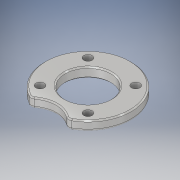
# Autodesk Inventor part: Motor Mount
Saved by Autodesk Inventor 2019.4 (Build 234330000, 330)
## iProperties
Created: 2019-03-01
Part Number: Motor Mount
Material: Aluminum 6061-AHC
Document SubType Name: Modeling
Designer: Petar
Density: 2.7 g/cm^3
Appearance: Aluminum - Dark
Mass: 6.25091 g
Surface Area: 19.0882 cm^2
Volume: 2.31515 cm^3
Author: Petar
Autodesk Inventor part; units mm, degrees
ref_plane "YZ Plane" through (0, 0, 0) normal (1, 0, 0) x (0, 1, 0)
ref_plane "XZ Plane" through (0, 0, 0) normal (0, 1, 0) x (-1, 0, 0)
ref_plane "XY Plane" through (0, 0, 0) normal (0, 0, 1) x (1, 0, 0)
sketch "Sketch1" plane through (0, 0, 0) normal (0, 1, 0) x (-1, 0, 0)
  circle A0 centre (0, 0) radius 9.25
  circle A1 centre (0, 0) radius 13.75 construction
  circle A2 centre (9.7227, -9.7227) radius 1.7
  line L0 (9.7227, -9.7227) -> (0, 0) construction
  circle A3 centre (9.7227, 9.7227) radius 1.7
  circle A4 centre (-9.7227, 9.7227) radius 1.7
  circle A5 centre (-9.7227, -9.7227) radius 1.7
  line L1 (0, 0) -> (0, -13.75) construction
  circle A6 centre (0, 0) radius 17.5
  circle A7 centre (0, 0) radius 10 construction
  line L2 (7.5, 15.8114) -> (0, 10) construction
  line L3 (0, 10) -> (-7.5, 15.8114) construction
  spline S0 degree 2 poles (7.5, 15.8114) (0, 10) (-7.5, 15.8114) knots 1 1 1 2 2 2
  line L4 (7.5, 15.8114) -> (-7.5, 15.8114) construction
  line L5 (0, 10) -> (0, 10) construction
  dimension "d10" = 20
  dimension "d0" = 18.5
  dimension "d2" = 3.4
  dimension "d6" = 360
  dimension "d8" = 45
  dimension "d11" = 15
  dimension "d27" = 0
  dimension "d30" = 7.5
  dimension "d31" = 3.75
  constraints: 8 end point, 7 centre point, 5 coincident, 5 point on circle, 2 vertical, 1 collinear, 1 horizontal, 1 vertical alignment, 15 other
  measures "d0" diameter of A0
  measures "d2" diameter of A2
  measures "d8" angle of L1 L0
  measures "d11" distance of L2.start L4.end
  measures "d27" distance of L5.start L5.end
extrude "Extrusion1" add sketch "Sketch1" along normal blind 4 contours A6 S0 picked at (12.2421, 4.8172)
fillet "Fillet1" radius 2 2 edges at (-7.5, 2, 15.8114) (7.5, 2, 15.8114)
fillet "Fillet2" radius 1 4 edges at (-7.5963, 0, 15.4658) (0, 0, 12.9057) (7.5963, 0, 15.4658) (0, 0, -17.5)
chamfer "Chamfer1" distance 0.5 angle 45 2 edges at (9.25, 4, 0) (9.25, 0, 0)
chamfer "Chamfer2" distance 0.5 angle 45 4 edges at (0, 4, -17.5) (-7.5963, 4, 15.4658) (0, 4, 12.9057) (7.5963, 4, 15.4658)
body "Solid1"
